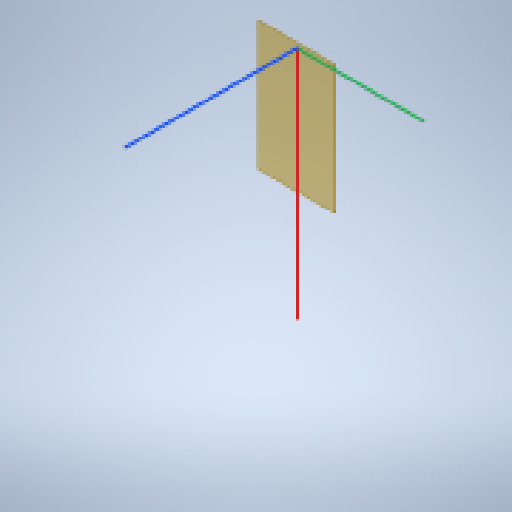
# Autodesk Inventor part: соси
Saved by Autodesk Inventor 2024.2 (Build 282272000, 272)
## iProperties
Created: 2026-05-04
Part Number: соси
Material: Типовые
Document SubType Name: Modeling
Designer: katya_notebook
Density: 1 g/cm^3
Appearance: По умолчанию
Author: katya_notebook
Autodesk Inventor part; units mm, degrees
ref_plane "YZ Plane" through (0, 0, 0) normal (1, 0, 0) x (0, 1, 0)
ref_plane "XZ Plane" through (0, 0, 0) normal (0, 1, 0) x (-1, 0, 0)
ref_plane "XY Plane" through (0, 0, 0) normal (0, 0, 1) x (1, 0, 0)
ref_plane "РабПлоскость1" through (0, 0, 0) normal (0, 0, 1) x (1, 0, 0)
sketch "Эскиз1" plane through (0, 0, 0) normal (0, 0, 1) x (1, 0, 0)
  line L0 (-0.8, 15.9546) -> (-0.8, 80.9546)
  line L1 (0.8, 15.9546) -> (0.8, 80.9546)
  line L2 (0.8, 80.9546) -> (-0.8, 80.9546)
  line L3 (-0.8, 15.9546) -> (0.8, 15.9546)
  line L4 (0.8, 15.9546) -> (0.8, -241.8245)
  line L5 (0.8, -241.8245) -> (-0.8, -241.8245)
  line L6 (-0.8, -241.8245) -> (-0.8, 15.9546)
  point P0 (0, 0)
  constraints: 14 end point, 2 horizontal, 2 parallel, 2 vertical, 1 collinear, 1 perpendicular, 4 other
revolve "Вращение1" add sketch "Эскиз1" angle 360 about axis through (0.8, 15.9546, 0) along (0, 1, 0)
ref_plane "РабПлоскость2" through (0, 0, 0) normal (0, 0, 1) x (1, 0, 0)
sketch "Эскиз2" plane through (0, 0, 0) normal (0, 0, 1) x (1, 0, 0)
  line L0 (-0.8, 84.1546) -> (176.9869, 84.1546)
  line L1 (176.9869, 84.1546) -> (176.9869, 80.9546)
  line L2 (176.9869, 80.9546) -> (-0.8, 80.9546)
  line L3 (-0.8, 80.9546) -> (-0.8, 84.1546)
  line L4 (2.4, -241.8245) -> (-0.8, -241.8245) projected
  line L5 (2.4, 80.9546) -> (-0.8, 80.9546) projected
  line L6 (-0.8, 82.5546) -> (176.9869, 82.5546)
  point P0 (0, 0)
  dimension "d1" = 3.2
  constraints: 10 end point, 2 midpoint, 2 parallel, 1 horizontal, 1 perpendicular
  measures "d1" distance between parallel lines of L2 L0
revolve "Вращение2" add sketch "Эскиз2" angle 360 about axis through (-0.8, 82.5546, 0) along (1, 0, 0) contours L6 L1 L2 L3
ref_plane "РабПлоскость3" through (0, 0, 0) normal (0, 0, 1) x (1, 0, 0)
sketch "Эскиз3" plane through (0, 0, 0) normal (0, 0, 1) x (1, 0, 0)
  circle A0 centre (0.807, 82.7995) radius 1.6
  point P0 (0, 0)
  dimension "d3" = 3.2
  constraints: 1 centre point
  measures "d3" diameter of A0
extrude "Выдавливание1" add sketch "Эскиз3" along normal blind 239
